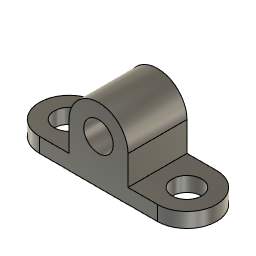
Lab#3.3 (Autodesk Fusion 360 design; units mm, degrees)
Autodesk Fusion 360 part; units mm, degrees
sketch "Horizontal" plane through (0, 0, 0) normal (0, 0, 1) x (1, 0, 0)
  line L0 (40, -20) -> (-40, -20)
  line L1 (-40, 20) -> (40, 20)
  circle A0 centre (40, 0) radius 10
  circle A1 centre (-40, 0) radius 10
  line L2 (20, 0) -> (40, 0) construction
  arc A2 (-40, 20) -> (-40, -20) centre (-40, 0) ccw
  arc A3 (40, -20) -> (40, 20) centre (40, 0) ccw
  dimension "d1" = 80
  dimension "d2" = 40
  dimension "d5" = 40
  dimension "d6" = 40
  constraint horizontal L0
  constraint parallel L0 L1
  constraint coincident A0.centre L2.end
  measures "d1" distance of L1.start L1.end
  measures "d2" distance of L0.end L1.start
  measures "d5" diameter of A2
  measures "d6" diameter of A3
extrude "Extrude1" add sketch "Horizontal" along normal blind 10
sketch "Vertical" plane through (0, 0, 0) normal (0, 1, 0) x (1, 0, 0)
  line L0 (-20, 0.0761) -> (20, 0.0761)
  line L1 (20, 0.0761) -> (20, -29.9239)
  line L2 (-10, -29.9239) -> (-20, -29.9239)
  line L3 (-20, -29.9239) -> (-20, 0.0761)
  line L4 (-40, 0) -> (-40, -10)
  circle A0 centre (0, -29.9239) radius 10
  arc A1 (-20, -29.9239) -> (20, -29.9239) centre (0, -29.9239) ccw
  dimension "d11" = 40
  dimension "d12" = 30
  dimension "d13" = 20
  dimension "d14" = 20
  dimension "d15" = 20
  constraint horizontal L0
  constraint vertical L1
  constraint horizontal L2
  constraint vertical L3
  constraint concentric A0 A1
  constraint coincident L2 A0.centre
  constraint coincident A0 L2.start
  measures "d11" distance of L0.start L0.end
  measures "d12" distance of L0.start L2.end
  measures "d13" distance of L3 L4
  measures "d14" radius of A1
  measures "d15" diameter of A0
extrude "Extrude2" add sketch "Vertical" along normal mid plane 40
named bodies: "Lab#3.3"
